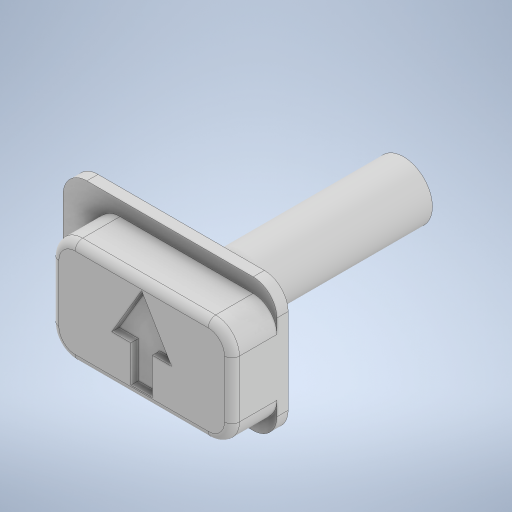
# Autodesk Inventor part: Button Cover
Saved by Autodesk Inventor 2023 (Build 270158000, 158)
## iProperties
Created: 2024-03-21
Part Number: Button Cover
Material: Generic
Document SubType Name: Modeling
Designer: Pobe Tran
Density: 1 g/cm^3
Appearance: Default
Author: Pobe Tran
Autodesk Inventor part; units mm, degrees
ref_plane "YZ Plane" through (0, 0, 0) normal (1, 0, 0) x (0, 1, 0)
ref_plane "XZ Plane" through (0, 0, 0) normal (0, 1, 0) x (-1, 0, 0)
ref_plane "XY Plane" through (0, 0, 0) normal (0, 0, 1) x (1, 0, 0)
sketch "Sketch1" plane through (0, 0, 0) normal (0, 0, 1) x (1, 0, 0)
  circle A0 centre (0, 0) radius 1.75 projected
  circle A1 centre (0, 0) radius 1.85
  circle A2 centre (0, 0) radius 3.85
  point P0 (0, 0)
  dimension "d0" = 0.1
  dimension "d1" = 2
  constraints: 2 centre point
  measures "d0" radial gap between concentric circles of A0 A1
  measures "d1" radial gap between concentric circles of A1 A2
extrude "Extrusion1" add sketch "Sketch1" against normal blind 5 contours A1 | A2
sketch "Sketch2" plane through (0, 0, 0) normal (0, 0, 1) x (1, 0, 0)
  point P0 (0, 0)
sketch "Sketch3" plane through (0, 0, 0) normal (0, 0, 1) x (1, 0, 0)
  circle A0 centre (0, 0) radius 3.85
  constraints: 1 centre point, 1 coincident
extrude "Extrusion2" add sketch "Sketch3" along normal blind 22.5
sketch "Sketch4" plane through (0, 0, 22.5) normal (0, 0, 1) x (1, 0, 0)
  line L0 (12.065, -6.985) -> (-12.065, -6.985)
  line L1 (-12.065, -6.985) -> (-12.065, 6.985)
  line L2 (-12.065, 6.985) -> (12.065, 6.985)
  line L3 (12.065, 6.985) -> (12.065, -6.985)
  circle A0 centre (0, 0) radius 1.85 projected
  line L4 (12.065, -6.985) -> (-12.065, 6.985) construction
  line L5 (-12.065, -6.985) -> (12.065, 6.985) construction
  line L6 (12.065, 12.065) -> (-12.065, 12.065) construction
  line L7 (-12.065, 12.065) -> (-12.065, 26.035) construction
  line L8 (-12.065, 26.035) -> (12.065, 26.035) construction
  line L9 (12.065, 26.035) -> (12.065, 12.065) construction
  line L10 (12.065, 12.065) -> (-12.065, 26.035) construction
  line L11 (-12.065, 12.065) -> (12.065, 26.035) construction
  line L12 (12.065, -8.89) -> (-16.51, -8.89)
  line L13 (-16.51, -8.89) -> (-16.51, 8.89)
  line L14 (-16.51, 8.89) -> (12.065, 8.89)
  line L15 (16.51, -8.89) -> (-16.51, 8.89) construction
  line L16 (-16.51, -8.89) -> (12.065, 6.4965) construction
  line L17 (12.065, -8.89) -> (12.065, 8.89)
  point P0 (0, 0)
  point P1 (0, 19.05)
  dimension "d6" = 24.13
  dimension "d7" = 13.97
  dimension "d10" = 19.05
  dimension "d16" = 17.78
  constraints: 36 end point, 3 midpoint, 3 parallel, 3 perpendicular, 2 horizontal, 2 point on line, 1 collinear, 1 vertical, 10 other
  measures "d6" distance of L1.end L2.end
  measures "d7" distance of L0.end L1.end
  measures "d10" distance of L0.start L6.start
  measures "d16" distance of L12.end L13.end
extrude "Extrusion3" add sketch "Sketch4" along normal blind 1.5 contours L17 L12 L13 L14 L2 L1 L0 | L0 L1 L2 L3 | A0
extrude "Extrusion4" add sketch "Sketch4" along normal blind 7.5 contours L0 L1 L2 L3 | A0
fillet "Fillet1" radius 3.175 8 edges at (-12.065, 6.985, 27) (12.065, 6.985, 27) (12.065, -6.985, 27) (-12.065, -6.985, 27) (-16.51, -8.89, 23.25) (12.065, 8.89, 23.25) (-16.51, 8.89, 23.25) (12.065, -8.89, 23.25)
sketch "Sketch5" plane through (0, 0, 30) normal (0, 0, 1) x (1, 0, 0)
  line L0 (0, 5.8462) -> (-3.9945, -0.9035)
  line L1 (3.9945, -0.9035) -> (0, 5.8462)
  line L2 (1.4311, -0.9035) -> (1.4311, -5.8047)
  line L3 (1.4311, -5.8047) -> (-1.4311, -5.8047)
  line L4 (-1.4311, -5.8047) -> (-1.4311, -0.9035)
  line L5 (8.89, 6.985) -> (-8.89, 6.985)
  arc A0 (8.89, -6.985) -> (12.065, -3.81) centre (8.89, -3.81) ccw
  line L6 (-8.89, -6.985) -> (8.89, -6.985)
  arc A1 (-12.065, -3.81) -> (-8.89, -6.985) centre (-8.89, -3.81) ccw
  arc A2 (-8.89, 6.985) -> (-12.065, 3.81) centre (-8.89, 3.81) ccw
  line L7 (-12.065, 3.81) -> (-12.065, -3.81)
  arc A3 (12.065, 3.81) -> (8.89, 6.985) centre (8.89, 3.81) ccw
  line L8 (12.065, -3.81) -> (12.065, 3.81)
  line L9 (-3.9945, -0.9035) -> (-1.4311, -0.9035)
  line L10 (1.4311, -0.9035) -> (3.9945, -0.9035)
  point P0 (0, 0)
  point P1 (0, 0)
  point P2 (0, -0.9035)
  point P3 (0, 6.985)
  constraints: 22 end point, 8 point on circle, 4 centre point, 1 equal length, 1 midpoint, 1 parallel
emboss "Emboss1" sketch "Sketch5" operation cut depth 1 direction (0, 0, -1) contours L1 L10 L2 L3 L4 L9 L0
fillet "Fillet2" radius 1 8 edges at (-11.1351, 6.0551, 30) (-12.065, 0, 30) (-11.1351, -6.0551, 30) (0, -6.985, 30) (11.1351, -6.0551, 30) (12.065, 0, 30) (11.1351, 6.0551, 30) (0, 6.985, 30)
body "Solid1"
